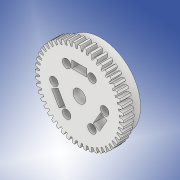
# Autodesk Inventor part: WA002
Saved by Autodesk Inventor 2017 SP1 (Build 210196100, 196)
## iProperties
Created: 2017-08-01
Part Number: WA002
Material: ABS Plastic
Document SubType Name: Modeling
Designer: Zach
Density: 1.06 g/cm^3
Appearance: CR White
Author: Zach
Autodesk Inventor part; units mm, degrees
ref_plane "YZ Plane" through (0, 0, 0) normal (1, 0, 0) x (0, 1, 0)
ref_plane "XZ Plane" through (0, 0, 0) normal (0, 1, 0) x (-1, 0, 0)
ref_plane "XY Plane" through (0, 0, 0) normal (0, 0, 1) x (1, 0, 0)
sketch "Sketch1" plane through (0, 0, 0) normal (0, 0, 1) x (1, 0, 0)
  circle A0 centre (0, 0) radius 6
  circle A1 centre (0, 0) radius 37.5
  dimension "d0" = 12
  dimension "d1" = 75
  constraints: 2 centre point, 2 coincident
  measures "d0" diameter of A0
  measures "d1" diameter of A1
extrude "Extrusion1" add sketch "Sketch1" along normal blind 10
sketch "Sketch2" plane through (0, 0, 10) normal (0, 0, 1) x (1, 0, 0)
  circle A0 centre (23.8125, 0) radius 2.5
  circle A1 centre (11.9063, 20.6222) radius 2.5
  circle A2 centre (-11.9062, 20.6222) radius 2.5
  circle A3 centre (-23.8125, 0) radius 2.5
  circle A4 centre (-11.9063, -20.6222) radius 2.5
  circle A5 centre (11.9062, -20.6222) radius 2.5
  point P0 (0, 0)
  dimension "d4" = 5
  dimension "d5" = 23.8125
  dimension "d8" = 360
  constraints: 6 centre point, 1 horizontal alignment, 13 other
  measures "d4" diameter of A0
  measures "d5" distance of A0.centre point (0, 0)
extrude "Extrusion2" cut sketch "Sketch2" against normal through all
sketch "Sketch3" plane through (0, 0, 10) normal (0, 0, 1) x (1, 0, 0)
  line L0 (7, 19) -> (-7, 19)
  line L1 (-7, 19) -> (-7, 26)
  line L2 (-7, 26) -> (7, 26)
  line L3 (7, 26) -> (7, 19)
  line L4 (-19.9545, -3.4378) -> (-12.9545, -15.5622)
  line L5 (-12.9545, -15.5622) -> (-19.0167, -19.0622)
  line L6 (-19.0167, -19.0622) -> (-26.0167, -6.9378)
  line L7 (-26.0167, -6.9378) -> (-19.9545, -3.4378)
  line L8 (12.9545, -15.5622) -> (19.9545, -3.4378)
  line L9 (19.9545, -3.4378) -> (26.0167, -6.9378)
  line L10 (26.0167, -6.9378) -> (19.0167, -19.0622)
  line L11 (19.0167, -19.0622) -> (12.9545, -15.5622)
  point P0 (0, 0)
  point P1 (0, 19)
  point P2 (-16.4545, -9.5)
  point P3 (16.4545, -9.5)
  dimension "d12" = 14
  dimension "d13" = 7
  dimension "d14" = 19
  dimension "d17" = 360
  constraints: 24 end point, 2 parallel, 1 horizontal, 1 midpoint, 1 perpendicular, 1 vertical alignment, 28 other
  measures "d12" distance of L1.end L2.end
  measures "d13" distance of L0.end L1.end
  measures "d14" distance from line of L0 point (0, 0)
extrude "Extrusion3" cut sketch "Sketch3" against normal blind 10
sketch "Sketch4" plane through (0, 0, 10) normal (0, 0, 1) x (1, 0, 0)
  circle A0 centre (0, 0) radius 37.5 projected
  circle A1 centre (0, 0) radius 37.5 projected
  arc A2 (41.4568, 1) -> (37.4568, 1.8) centre (36.5424, -13.1721) ccw
  arc A3 (41.4568, -1) -> (41.4568, 1) centre (21.4818, 0) ccw
  arc A4 (37.4568, -1.8) -> (41.4568, -1) centre (36.5424, 13.1721) ccw
  arc A5 (37.4568, -1.8) -> (37.4568, 1.8) centre (0, 0) ccw
  arc A6 (40.9716, 6.4026) -> (36.9014, 6.6737) centre (37.949, -8.2897) ccw
  arc A7 (37.3713, 3.1045) -> (36.9014, 6.6737) centre (0, 0) ccw
  arc A8 (37.3713, 3.1045) -> (41.2326, 4.4198) centre (34.5104, 17.8291) ccw
  arc A9 (41.2326, 4.4198) -> (40.9716, 6.4026) centre (21.298, 2.8039) ccw
  arc A10 (39.7854, 11.6957) -> (35.7146, 11.4332) centre (38.7064, -3.2654) ccw
  arc A11 (36.6463, 7.9559) -> (35.7146, 11.4332) centre (0, 0) ccw
  arc A12 (36.6463, 7.9559) -> (40.303, 9.7639) centre (31.888, 22.1811) ccw
  arc A13 (40.303, 9.7639) -> (39.7854, 11.6957) centre (20.7498, 5.5599) ccw
  arc A14 (37.9184, 16.7887) -> (33.9167, 15.9971) centre (38.8015, 1.8147) ccw
  arc A15 (35.2944, 12.6711) -> (33.9167, 15.9971) centre (0, 0) ccw
  arc A16 (35.2944, 12.6711) -> (38.6837, 14.9409) centre (28.72, 26.1536) ccw
  arc A17 (38.6837, 14.9409) -> (37.9184, 16.7887) centre (19.8466, 8.2207) ccw
  arc A18 (35.4026, 21.5944) -> (31.5385, 20.2872) centre (38.2327, 6.8638) ccw
  arc A19 (33.3385, 17.1695) -> (31.5385, 20.2872) centre (0, 0) ccw
  arc A20 (33.3385, 17.1695) -> (36.4026, 19.8624) centre (25.0606, 29.6786) ccw
  arc A21 (36.4026, 19.8624) -> (35.4026, 21.5944) centre (18.6038, 10.7409) ccw
  arc A22 (32.2811, 26.0306) -> (28.6207, 24.2303) centre (37.0097, 11.7954) ccw
  arc A23 (30.8122, 21.3742) -> (28.6207, 24.2303) centre (0, 0) ccw
  arc A24 (30.8122, 21.3742) -> (33.4986, 24.4439) centre (20.9723, 32.6957) ccw
  arc A25 (33.4986, 24.4439) -> (32.2811, 26.0306) centre (17.0427, 13.0773) ccw
  arc A26 (28.6073, 30.0215) -> (25.2131, 27.7587) centre (35.1534, 16.5253) ccw
  arc A27 (27.7587, 25.2131) -> (25.2131, 27.7587) centre (0, 0) ccw
  arc A28 (27.7587, 25.2131) -> (30.0215, 28.6073) centre (16.5253, 35.1534) ccw
  arc A29 (30.0215, 28.6073) -> (28.6073, 30.0215) centre (15.1899, 15.1899) ccw
  arc A30 (24.4439, 33.4986) -> (21.3742, 30.8122) centre (32.6957, 20.9723) ccw
  arc A31 (24.2303, 28.6207) -> (21.3742, 30.8122) centre (0, 0) ccw
  arc A32 (24.2303, 28.6207) -> (26.0306, 32.2811) centre (11.7954, 37.0097) ccw
  arc A33 (26.0306, 32.2811) -> (24.4439, 33.4986) centre (13.0773, 17.0427) ccw
  arc A34 (19.8624, 36.4026) -> (17.1695, 33.3385) centre (29.6786, 25.0606) ccw
  arc A35 (20.2872, 31.5385) -> (17.1695, 33.3385) centre (0, 0) ccw
  arc A36 (20.2872, 31.5385) -> (21.5944, 35.4026) centre (6.8638, 38.2327) ccw
  arc A37 (21.5944, 35.4026) -> (19.8624, 36.4026) centre (10.7409, 18.6038) ccw
  arc A38 (14.9409, 38.6837) -> (12.6711, 35.2944) centre (26.1536, 28.72) ccw
  arc A39 (15.9971, 33.9167) -> (12.6711, 35.2944) centre (0, 0) ccw
  arc A40 (15.9971, 33.9167) -> (16.7887, 37.9184) centre (1.8147, 38.8015) ccw
  arc A41 (16.7887, 37.9184) -> (14.9409, 38.6837) centre (8.2207, 19.8466) ccw
  arc A42 (9.7639, 40.303) -> (7.9559, 36.6463) centre (22.1811, 31.888) ccw
  arc A43 (11.4332, 35.7146) -> (7.9559, 36.6463) centre (0, 0) ccw
  arc A44 (11.4332, 35.7146) -> (11.6957, 39.7854) centre (-3.2654, 38.7064) ccw
  arc A45 (11.6957, 39.7854) -> (9.7639, 40.303) centre (5.5599, 20.7498) ccw
  arc A46 (4.4198, 41.2326) -> (3.1045, 37.3713) centre (17.8291, 34.5104) ccw
  arc A47 (6.6737, 36.9014) -> (3.1045, 37.3713) centre (0, 0) ccw
  arc A48 (6.6737, 36.9014) -> (6.4026, 40.9716) centre (-8.2897, 37.949) ccw
  arc A49 (6.4026, 40.9716) -> (4.4198, 41.2326) centre (2.8039, 21.298) ccw
  arc A50 (-1, 41.4568) -> (-1.8, 37.4568) centre (13.1721, 36.5424) ccw
  arc A51 (1.8, 37.4568) -> (-1.8, 37.4568) centre (0, 0) ccw
  arc A52 (1.8, 37.4568) -> (1, 41.4568) centre (-13.1721, 36.5424) ccw
  arc A53 (1, 41.4568) -> (-1, 41.4568) centre (0, 21.4818) ccw
  arc A54 (-6.4026, 40.9716) -> (-6.6737, 36.9014) centre (8.2897, 37.949) ccw
  arc A55 (-3.1045, 37.3713) -> (-6.6737, 36.9014) centre (0, 0) ccw
  arc A56 (-3.1045, 37.3713) -> (-4.4198, 41.2326) centre (-17.8291, 34.5104) ccw
  arc A57 (-4.4198, 41.2326) -> (-6.4026, 40.9716) centre (-2.8039, 21.298) ccw
  arc A58 (-11.6957, 39.7854) -> (-11.4332, 35.7146) centre (3.2654, 38.7064) ccw
  arc A59 (-7.9559, 36.6463) -> (-11.4332, 35.7146) centre (0, 0) ccw
  arc A60 (-7.9559, 36.6463) -> (-9.7639, 40.303) centre (-22.1811, 31.888) ccw
  arc A61 (-9.7639, 40.303) -> (-11.6957, 39.7854) centre (-5.5599, 20.7498) ccw
  arc A62 (-16.7887, 37.9184) -> (-15.9971, 33.9167) centre (-1.8147, 38.8015) ccw
  arc A63 (-12.6711, 35.2944) -> (-15.9971, 33.9167) centre (0, 0) ccw
  arc A64 (-12.6711, 35.2944) -> (-14.9409, 38.6837) centre (-26.1536, 28.72) ccw
  arc A65 (-14.9409, 38.6837) -> (-16.7887, 37.9184) centre (-8.2207, 19.8466) ccw
  arc A66 (-21.5944, 35.4026) -> (-20.2872, 31.5385) centre (-6.8638, 38.2327) ccw
  arc A67 (-17.1695, 33.3385) -> (-20.2872, 31.5385) centre (0, 0) ccw
  arc A68 (-17.1695, 33.3385) -> (-19.8624, 36.4026) centre (-29.6786, 25.0606) ccw
  arc A69 (-19.8624, 36.4026) -> (-21.5944, 35.4026) centre (-10.7409, 18.6038) ccw
  arc A70 (-26.0306, 32.2811) -> (-24.2303, 28.6207) centre (-11.7954, 37.0097) ccw
  arc A71 (-21.3742, 30.8122) -> (-24.2303, 28.6207) centre (0, 0) ccw
  arc A72 (-21.3742, 30.8122) -> (-24.4439, 33.4986) centre (-32.6957, 20.9723) ccw
  arc A73 (-24.4439, 33.4986) -> (-26.0306, 32.2811) centre (-13.0773, 17.0427) ccw
  arc A74 (-30.0215, 28.6073) -> (-27.7587, 25.2131) centre (-16.5253, 35.1534) ccw
  arc A75 (-25.2131, 27.7587) -> (-27.7587, 25.2131) centre (0, 0) ccw
  arc A76 (-25.2131, 27.7587) -> (-28.6073, 30.0215) centre (-35.1534, 16.5253) ccw
  arc A77 (-28.6073, 30.0215) -> (-30.0215, 28.6073) centre (-15.1899, 15.1899) ccw
  arc A78 (-33.4986, 24.4439) -> (-30.8122, 21.3742) centre (-20.9723, 32.6957) ccw
  arc A79 (-28.6207, 24.2303) -> (-30.8122, 21.3742) centre (0, 0) ccw
  arc A80 (-28.6207, 24.2303) -> (-32.2811, 26.0306) centre (-37.0097, 11.7954) ccw
  arc A81 (-32.2811, 26.0306) -> (-33.4986, 24.4439) centre (-17.0427, 13.0773) ccw
  arc A82 (-36.4026, 19.8624) -> (-33.3385, 17.1695) centre (-25.0606, 29.6786) ccw
  arc A83 (-31.5385, 20.2872) -> (-33.3385, 17.1695) centre (0, 0) ccw
  arc A84 (-31.5385, 20.2872) -> (-35.4026, 21.5944) centre (-38.2327, 6.8638) ccw
  arc A85 (-35.4026, 21.5944) -> (-36.4026, 19.8624) centre (-18.6038, 10.7409) ccw
  arc A86 (-38.6837, 14.9409) -> (-35.2944, 12.6711) centre (-28.72, 26.1536) ccw
  arc A87 (-33.9167, 15.9971) -> (-35.2944, 12.6711) centre (0, 0) ccw
  arc A88 (-33.9167, 15.9971) -> (-37.9184, 16.7887) centre (-38.8015, 1.8147) ccw
  arc A89 (-37.9184, 16.7887) -> (-38.6837, 14.9409) centre (-19.8466, 8.2207) ccw
  arc A90 (-40.303, 9.7639) -> (-36.6463, 7.9559) centre (-31.888, 22.1811) ccw
  arc A91 (-35.7146, 11.4332) -> (-36.6463, 7.9559) centre (0, 0) ccw
  arc A92 (-35.7146, 11.4332) -> (-39.7854, 11.6957) centre (-38.7064, -3.2654) ccw
  arc A93 (-39.7854, 11.6957) -> (-40.303, 9.7639) centre (-20.7498, 5.5599) ccw
  arc A94 (-41.2326, 4.4198) -> (-37.3713, 3.1045) centre (-34.5104, 17.8291) ccw
  arc A95 (-36.9014, 6.6737) -> (-37.3713, 3.1045) centre (0, 0) ccw
  arc A96 (-36.9014, 6.6737) -> (-40.9716, 6.4026) centre (-37.949, -8.2897) ccw
  arc A97 (-40.9716, 6.4026) -> (-41.2326, 4.4198) centre (-21.298, 2.8039) ccw
  arc A98 (-41.4568, -1) -> (-37.4568, -1.8) centre (-36.5424, 13.1721) ccw
  arc A99 (-37.4568, 1.8) -> (-37.4568, -1.8) centre (0, 0) ccw
  arc A100 (-37.4568, 1.8) -> (-41.4568, 1) centre (-36.5424, -13.1721) ccw
  arc A101 (-41.4568, 1) -> (-41.4568, -1) centre (-21.4818, 0) ccw
  arc A102 (-40.9716, -6.4026) -> (-36.9014, -6.6737) centre (-37.949, 8.2897) ccw
  arc A103 (-37.3713, -3.1045) -> (-36.9014, -6.6737) centre (0, 0) ccw
  arc A104 (-37.3713, -3.1045) -> (-41.2326, -4.4198) centre (-34.5104, -17.8291) ccw
  arc A105 (-41.2326, -4.4198) -> (-40.9716, -6.4026) centre (-21.298, -2.8039) ccw
  arc A106 (-39.7854, -11.6957) -> (-35.7146, -11.4332) centre (-38.7064, 3.2654) ccw
  arc A107 (-36.6463, -7.9559) -> (-35.7146, -11.4332) centre (0, 0) ccw
  arc A108 (-36.6463, -7.9559) -> (-40.303, -9.7639) centre (-31.888, -22.1811) ccw
  arc A109 (-40.303, -9.7639) -> (-39.7854, -11.6957) centre (-20.7498, -5.5599) ccw
  arc A110 (-37.9184, -16.7887) -> (-33.9167, -15.9971) centre (-38.8015, -1.8147) ccw
  arc A111 (-35.2944, -12.6711) -> (-33.9167, -15.9971) centre (0, 0) ccw
  arc A112 (-35.2944, -12.6711) -> (-38.6837, -14.9409) centre (-28.72, -26.1536) ccw
  arc A113 (-38.6837, -14.9409) -> (-37.9184, -16.7887) centre (-19.8466, -8.2207) ccw
  arc A114 (-35.4026, -21.5944) -> (-31.5385, -20.2872) centre (-38.2327, -6.8638) ccw
  arc A115 (-33.3385, -17.1695) -> (-31.5385, -20.2872) centre (0, 0) ccw
  arc A116 (-33.3385, -17.1695) -> (-36.4026, -19.8624) centre (-25.0606, -29.6786) ccw
  arc A117 (-36.4026, -19.8624) -> (-35.4026, -21.5944) centre (-18.6038, -10.7409) ccw
  arc A118 (-32.2811, -26.0306) -> (-28.6207, -24.2303) centre (-37.0097, -11.7954) ccw
  arc A119 (-30.8122, -21.3742) -> (-28.6207, -24.2303) centre (0, 0) ccw
  arc A120 (-30.8122, -21.3742) -> (-33.4986, -24.4439) centre (-20.9723, -32.6957) ccw
  arc A121 (-33.4986, -24.4439) -> (-32.2811, -26.0306) centre (-17.0427, -13.0773) ccw
  arc A122 (-28.6073, -30.0215) -> (-25.2131, -27.7587) centre (-35.1534, -16.5253) ccw
  arc A123 (-27.7587, -25.2131) -> (-25.2131, -27.7587) centre (0, 0) ccw
  arc A124 (-27.7587, -25.2131) -> (-30.0215, -28.6073) centre (-16.5253, -35.1534) ccw
  arc A125 (-30.0215, -28.6073) -> (-28.6073, -30.0215) centre (-15.1899, -15.1899) ccw
  arc A126 (-24.4439, -33.4986) -> (-21.3742, -30.8122) centre (-32.6957, -20.9723) ccw
  arc A127 (-24.2303, -28.6207) -> (-21.3742, -30.8122) centre (0, 0) ccw
  arc A128 (-24.2303, -28.6207) -> (-26.0306, -32.2811) centre (-11.7954, -37.0097) ccw
  arc A129 (-26.0306, -32.2811) -> (-24.4439, -33.4986) centre (-13.0773, -17.0427) ccw
  arc A130 (-19.8624, -36.4026) -> (-17.1695, -33.3385) centre (-29.6786, -25.0606) ccw
  arc A131 (-20.2872, -31.5385) -> (-17.1695, -33.3385) centre (0, 0) ccw
  arc A132 (-20.2872, -31.5385) -> (-21.5944, -35.4026) centre (-6.8638, -38.2327) ccw
  arc A133 (-21.5944, -35.4026) -> (-19.8624, -36.4026) centre (-10.7409, -18.6038) ccw
  arc A134 (-14.9409, -38.6837) -> (-12.6711, -35.2944) centre (-26.1536, -28.72) ccw
  arc A135 (-15.9971, -33.9167) -> (-12.6711, -35.2944) centre (0, 0) ccw
  arc A136 (-15.9971, -33.9167) -> (-16.7887, -37.9184) centre (-1.8147, -38.8015) ccw
  arc A137 (-16.7887, -37.9184) -> (-14.9409, -38.6837) centre (-8.2207, -19.8466) ccw
  arc A138 (-9.7639, -40.303) -> (-7.9559, -36.6463) centre (-22.1811, -31.888) ccw
  arc A139 (-11.4332, -35.7146) -> (-7.9559, -36.6463) centre (0, 0) ccw
  arc A140 (-11.4332, -35.7146) -> (-11.6957, -39.7854) centre (3.2654, -38.7064) ccw
  arc A141 (-11.6957, -39.7854) -> (-9.7639, -40.303) centre (-5.5599, -20.7498) ccw
  arc A142 (-4.4198, -41.2326) -> (-3.1045, -37.3713) centre (-17.8291, -34.5104) ccw
  arc A143 (-6.6737, -36.9014) -> (-3.1045, -37.3713) centre (0, 0) ccw
  arc A144 (-6.6737, -36.9014) -> (-6.4026, -40.9716) centre (8.2897, -37.949) ccw
  arc A145 (-6.4026, -40.9716) -> (-4.4198, -41.2326) centre (-2.8039, -21.298) ccw
  arc A146 (1, -41.4568) -> (1.8, -37.4568) centre (-13.1721, -36.5424) ccw
  arc A147 (-1.8, -37.4568) -> (1.8, -37.4568) centre (0, 0) ccw
  arc A148 (-1.8, -37.4568) -> (-1, -41.4568) centre (13.1721, -36.5424) ccw
  arc A149 (-1, -41.4568) -> (1, -41.4568) centre (0, -21.4818) ccw
  arc A150 (6.4026, -40.9716) -> (6.6737, -36.9014) centre (-8.2897, -37.949) ccw
  arc A151 (3.1045, -37.3713) -> (6.6737, -36.9014) centre (0, 0) ccw
  arc A152 (3.1045, -37.3713) -> (4.4198, -41.2326) centre (17.8291, -34.5104) ccw
  arc A153 (4.4198, -41.2326) -> (6.4026, -40.9716) centre (2.8039, -21.298) ccw
  arc A154 (11.6957, -39.7854) -> (11.4332, -35.7146) centre (-3.2654, -38.7064) ccw
  arc A155 (7.9559, -36.6463) -> (11.4332, -35.7146) centre (0, 0) ccw
  arc A156 (7.9559, -36.6463) -> (9.7639, -40.303) centre (22.1811, -31.888) ccw
  arc A157 (9.7639, -40.303) -> (11.6957, -39.7854) centre (5.5599, -20.7498) ccw
  arc A158 (16.7887, -37.9184) -> (15.9971, -33.9167) centre (1.8147, -38.8015) ccw
  arc A159 (12.6711, -35.2944) -> (15.9971, -33.9167) centre (0, 0) ccw
  arc A160 (12.6711, -35.2944) -> (14.9409, -38.6837) centre (26.1536, -28.72) ccw
  arc A161 (14.9409, -38.6837) -> (16.7887, -37.9184) centre (8.2207, -19.8466) ccw
  arc A162 (21.5944, -35.4026) -> (20.2872, -31.5385) centre (6.8638, -38.2327) ccw
  arc A163 (17.1695, -33.3385) -> (20.2872, -31.5385) centre (0, 0) ccw
  arc A164 (17.1695, -33.3385) -> (19.8624, -36.4026) centre (29.6786, -25.0606) ccw
  arc A165 (19.8624, -36.4026) -> (21.5944, -35.4026) centre (10.7409, -18.6038) ccw
  arc A166 (26.0306, -32.2811) -> (24.2303, -28.6207) centre (11.7954, -37.0097) ccw
  arc A167 (21.3742, -30.8122) -> (24.2303, -28.6207) centre (0, 0) ccw
  arc A168 (21.3742, -30.8122) -> (24.4439, -33.4986) centre (32.6957, -20.9723) ccw
  arc A169 (24.4439, -33.4986) -> (26.0306, -32.2811) centre (13.0773, -17.0427) ccw
  arc A170 (30.0215, -28.6073) -> (27.7587, -25.2131) centre (16.5253, -35.1534) ccw
  arc A171 (25.2131, -27.7587) -> (27.7587, -25.2131) centre (0, 0) ccw
  arc A172 (25.2131, -27.7587) -> (28.6073, -30.0215) centre (35.1534, -16.5253) ccw
  arc A173 (28.6073, -30.0215) -> (30.0215, -28.6073) centre (15.1899, -15.1899) ccw
  arc A174 (33.4986, -24.4439) -> (30.8122, -21.3742) centre (20.9723, -32.6957) ccw
  arc A175 (28.6207, -24.2303) -> (30.8122, -21.3742) centre (0, 0) ccw
  arc A176 (28.6207, -24.2303) -> (32.2811, -26.0306) centre (37.0097, -11.7954) ccw
  arc A177 (32.2811, -26.0306) -> (33.4986, -24.4439) centre (17.0427, -13.0773) ccw
  arc A178 (36.4026, -19.8624) -> (33.3385, -17.1695) centre (25.0606, -29.6786) ccw
  arc A179 (31.5385, -20.2872) -> (33.3385, -17.1695) centre (0, 0) ccw
  arc A180 (31.5385, -20.2872) -> (35.4026, -21.5944) centre (38.2327, -6.8638) ccw
  arc A181 (35.4026, -21.5944) -> (36.4026, -19.8624) centre (18.6038, -10.7409) ccw
  arc A182 (38.6837, -14.9409) -> (35.2944, -12.6711) centre (28.72, -26.1536) ccw
  arc A183 (33.9167, -15.9971) -> (35.2944, -12.6711) centre (0, 0) ccw
  arc A184 (33.9167, -15.9971) -> (37.9184, -16.7887) centre (38.8015, -1.8147) ccw
  arc A185 (37.9184, -16.7887) -> (38.6837, -14.9409) centre (19.8466, -8.2207) ccw
  arc A186 (40.303, -9.7639) -> (36.6463, -7.9559) centre (31.888, -22.1811) ccw
  arc A187 (35.7146, -11.4332) -> (36.6463, -7.9559) centre (0, 0) ccw
  arc A188 (35.7146, -11.4332) -> (39.7854, -11.6957) centre (38.7064, 3.2654) ccw
  arc A189 (39.7854, -11.6957) -> (40.303, -9.7639) centre (20.7498, -5.5599) ccw
  arc A190 (41.2326, -4.4198) -> (37.3713, -3.1045) centre (34.5104, -17.8291) ccw
  arc A191 (36.9014, -6.6737) -> (37.3713, -3.1045) centre (0, 0) ccw
  arc A192 (36.9014, -6.6737) -> (40.9716, -6.4026) centre (37.949, 8.2897) ccw
  arc A193 (40.9716, -6.4026) -> (41.2326, -4.4198) centre (21.298, -2.8039) ccw
  line L0 (-26.0167, -6.9378) -> (-19.9545, -3.4378) projected
  line L1 (-19.9545, -3.4378) -> (-12.9545, -15.5622) projected
  line L2 (-12.9545, -15.5622) -> (-19.0167, -19.0622) projected
  line L3 (-19.0167, -19.0622) -> (-26.0167, -6.9378) projected
  line L4 (7, 26) -> (7, 19) projected
  line L5 (7, 19) -> (-7, 19) projected
  line L6 (-7, 19) -> (-7, 26) projected
  line L7 (-7, 26) -> (7, 26) projected
  line L8 (19.0167, -19.0622) -> (12.9545, -15.5622) projected
  line L9 (12.9545, -15.5622) -> (19.9545, -3.4378) projected
  line L10 (19.9545, -3.4378) -> (26.0167, -6.9378) projected
  line L11 (26.0167, -6.9378) -> (19.0167, -19.0622) projected
  circle A194 centre (-11.9063, -20.6222) radius 2.5 projected
  circle A195 centre (-11.9062, 20.6222) radius 2.5 projected
  circle A196 centre (23.8125, 0) radius 2.5 projected
  circle A197 centre (11.9063, 20.6222) radius 2.5 projected
  circle A198 centre (-23.8125, 0) radius 2.5 projected
  circle A199 centre (11.9062, -20.6222) radius 2.5 projected
  circle A200 centre (0, 0) radius 6 projected
  circle A201 centre (0, 0) radius 37.5 projected
  point P0 (41.4818, 0)
  point P1 (41.1269, 5.4145)
  point P2 (40.0683, 10.7363)
  point P3 (38.3242, 15.8744)
  point P4 (35.9243, 20.7409)
  point P5 (32.9097, 25.2525)
  point P6 (29.3321, 29.3321)
  point P7 (25.2525, 32.9097)
  point P8 (20.7409, 35.9243)
  point P9 (15.8744, 38.3242)
  point P10 (10.7363, 40.0683)
  point P11 (5.4145, 41.1269)
  point P12 (0, 41.4818)
  point P13 (-5.4145, 41.1269)
  point P14 (-10.7363, 40.0683)
  point P15 (-15.8744, 38.3242)
  point P16 (-20.7409, 35.9243)
  point P17 (-25.2525, 32.9097)
  point P18 (-29.3321, 29.3321)
  point P19 (-32.9097, 25.2525)
  point P20 (-35.9243, 20.7409)
  point P21 (-38.3242, 15.8744)
  point P22 (-40.0683, 10.7363)
  point P23 (-41.1269, 5.4145)
  point P24 (-41.4818, 0)
  point P25 (-41.1269, -5.4145)
  point P26 (-40.0683, -10.7363)
  point P27 (-38.3242, -15.8744)
  point P28 (-35.9243, -20.7409)
  point P29 (-32.9097, -25.2525)
  point P30 (-29.3321, -29.3321)
  point P31 (-25.2525, -32.9097)
  point P32 (-20.7409, -35.9243)
  point P33 (-15.8744, -38.3242)
  point P34 (-10.7363, -40.0683)
  point P35 (-5.4145, -41.1269)
  point P36 (0, -41.4818)
  point P37 (5.4145, -41.1269)
  point P38 (10.7363, -40.0683)
  point P39 (15.8744, -38.3242)
  point P40 (20.7409, -35.9243)
  point P41 (25.2525, -32.9097)
  point P42 (29.3321, -29.3321)
  point P43 (32.9097, -25.2525)
  point P44 (35.9243, -20.7409)
  point P45 (38.3242, -15.8744)
  point P46 (40.0683, -10.7363)
  point P47 (41.1269, -5.4145)
  dimension "d21" = 15
  dimension "d22" = 20
  dimension "d25" = 15
  dimension "d28" = 2
  dimension "d30" = 4
  dimension "d31" = 1.8
  dimension "d32" = 1.8
  dimension "d35" = 360
  constraints: 389 point on circle, 192 centre point, 1 concentric, 1 horizontal alignment, 1 vertical alignment, 625 other
  measures "d21" radius of A2
  measures "d22" radius of A3
  measures "d25" radius of A4
  measures "d28" distance of A3.start A2.start
  measures "d30" horizontal distance of A0.start A2.start
  measures "d31" vertical distance of point (41.482, 0) A0.start
  measures "d32" vertical distance of point (41.482, 0) A0.end
extrude "Extrusion4" add sketch "Sketch4" along normal blind 10
sketch "Sketch5" plane through (0, 0, 20) normal (0, 0, 1) x (1, 0, 0)
  circle A0 centre (23.8125, 0) radius 2.5 projected
  circle A1 centre (23.8125, 0) radius 4
  circle A2 centre (11.9063, 20.6222) radius 4
  circle A3 centre (-11.9062, 20.6222) radius 4
  circle A4 centre (-23.8125, 0) radius 4
  circle A5 centre (-11.9063, -20.6222) radius 4
  circle A6 centre (11.9062, -20.6222) radius 4
  point P0 (0, 0)
  dimension "d39" = 8
  dimension "d42" = 360
  constraints: 6 centre point, 1 coincident, 13 other
  measures "d39" diameter of A1
extrude "Extrusion5" cut sketch "Sketch5" against normal blind 10 contours A0 | A1 | A2 | A3 | A4 | A5 | A6
body "Solid1"
